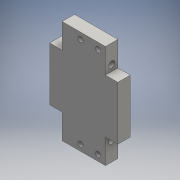
# Autodesk Inventor part: frameBack
Saved by Autodesk Inventor 2016 (Build 200138000, 138)
## iProperties
Created: 2016-05-21
Part Number: frameBack
Material: Generic
Document SubType Name: Modeling
Designer: Henrik Samuelsson
Density: 1 g/cm^3
Appearance: Default
Author: Henrik Samuelsson
Autodesk Inventor part; units mm, degrees
ref_plane "YZ Plane" through (0, 0, 0) normal (1, 0, 0) x (0, 1, 0)
ref_plane "XZ Plane" through (0, 0, 0) normal (0, 1, 0) x (-1, 0, 0)
ref_plane "XY Plane" through (0, 0, 0) normal (0, 0, 1) x (1, 0, 0)
sketch "Sketch1" plane through (0, 0, 0) normal (0, 1, 0) x (-1, 0, 0)
  line L0 (0, 0) -> (66, 0)
  line L1 (66, 0) -> (66, -100)
  line L2 (66, -100) -> (0, -100)
  line L3 (0, -100) -> (0, 0)
  line L4 (66, 0) -> (54, 0)
  line L5 (54, 0) -> (54, -12)
  line L6 (54, -12) -> (66, -12)
  line L7 (66, -12) -> (66, 0)
  line L8 (0, 0) -> (12, 0)
  line L9 (12, 0) -> (12, -12)
  line L10 (12, -12) -> (0, -12)
  line L11 (0, -12) -> (0, 0)
  line L12 (0, -100) -> (12, -100)
  line L13 (12, -100) -> (12, -88)
  line L14 (12, -88) -> (0, -88)
  line L15 (0, -88) -> (0, -100)
  line L16 (66, -100) -> (54, -100)
  line L17 (54, -100) -> (54, -88)
  line L18 (54, -88) -> (66, -88)
  line L19 (66, -88) -> (66, -100)
  dimension "d0" = 66
  dimension "d1" = 100
  dimension "d2" = 12
  dimension "d3" = 12
  dimension "d4" = 12
  dimension "d5" = 12
  dimension "d6" = 12
  dimension "d7" = 12
  dimension "d8" = 12
  dimension "d9" = 12
  constraints: 40 end point, 10 parallel, 5 horizontal, 5 perpendicular
  measures "d0" distance of L1.end L2.end
  measures "d1" distance of L0.end L1.end
  measures "d2" distance of L6.end L5.end
  measures "d3" distance of L5.end L4.end
  measures "d4" distance of L9.end L10.end
  measures "d5" distance of L8.end L9.end
  measures "d6" distance of L14.end L13.end
  measures "d7" distance of L13.end L12.end
  measures "d8" distance of L17.end L18.end
  measures "d9" distance of L16.end L17.end
extrude "Extrusion1" add sketch "Sketch1" along normal blind 12 contours L0 L5 L6 L1 L18 L17 L2 L13 L14 L3 L10 L9
sketch "Sketch5" plane through (-66, 0, -88) normal (-1, 0, 0) x (0, 0, 1)
  line L0 (0, 12) -> (-12, 12) projected
  line L1 (0, 12) -> (12, 12)
  line L2 (12, 12) -> (12, 0)
  line L3 (12, 0) -> (0, 0)
  line L4 (0, 0) -> (0, 12)
  line L5 (76, 12) -> (64, 12)
  line L6 (64, 12) -> (64, 0)
  line L7 (64, 0) -> (76, 0)
  line L8 (76, 0) -> (76, 12)
  point P0 (88, 0)
  dimension "d42" = 12
  dimension "d43" = 12
  dimension "d44" = 12
  dimension "d45" = 12
  dimension "d46" = 12
  constraints: 16 end point, 4 parallel, 2 horizontal, 2 perpendicular, 1 point on line
  measures "d42" distance of L2.end L3.end
  measures "d43" distance of L1.end L2.end
  measures "d44" distance of L7.end L6.end
  measures "d45" distance of L6.end L5.end
  measures "d46" distance of L7.end point (88, 0)
extrude "Extrusion5" cut sketch "Sketch5" against normal blind 12
sketch "Sketch6" plane through (0, 0, -12) normal (1, 0, 0) x (0, 0, -1)
  line L0 (76, 0) -> (76, 12) projected
  line L1 (64, 12) -> (12, 12) projected
  line L2 (76, 0) -> (64, 0)
  line L3 (64, 0) -> (64, 12)
  line L4 (64, 12) -> (76, 12)
  line L5 (76, 12) -> (76, 0)
  line L6 (64, 0) -> (12, 0) projected
  line L7 (12, 12) -> (-12, 12) projected
  line L8 (0, 0) -> (12, 0)
  line L9 (12, 0) -> (12, 12)
  line L10 (12, 12) -> (0, 12)
  line L11 (0, 12) -> (0, 0)
  point P0 (-12, 0)
  dimension "d49" = 12
  dimension "d50" = 12
  constraints: 16 end point, 4 parallel, 2 horizontal, 2 perpendicular
  measures "d49" distance of L1.start L4.end
  measures "d50" distance of L2.end L1.start
extrude "Extrusion6" cut sketch "Sketch6" against normal blind 12 contours L2 L3 L4 L0 | L8 L11 L7 L9
sketch "Sketch7" plane through (-12, -12, -100) normal (1, 0, 0) x (0, 0, -1)
  circle A0 centre (-18, 18) radius 3
  circle A1 centre (-82, 18) radius 3
  line L0 (-100, 24) -> (-76, 24) projected
  line L1 (-76, 24) -> (-76, 12) projected
  line L2 (-24, 12) -> (-24, 24) projected
  line L3 (-24, 24) -> (0, 24) projected
  point P0 (-100, 12)
  dimension "d53" = 6
  dimension "d54" = 6
  dimension "d55" = 6
  dimension "d56" = 6
  dimension "d57" = 6
  dimension "d58" = 6
  constraints: 2 centre point
  measures "d53" diameter of A0
  measures "d54" diameter of A1
  measures "d55" distance from line of L0 A1.centre
  measures "d56" distance from line of L1 A1.centre
  measures "d57" distance from line of L2 A0.centre
  measures "d58" distance from line of L3 A0.centre
extrude "Extrusion7" cut sketch "Sketch7" against normal up to next
sketch "Sketch8" plane through (0, 0, 0) normal (0, -1, 0) x (1, 0, 0)
  circle A0 centre (-19, -6) radius 2.5
  circle A1 centre (-36, -6) radius 2.5
  circle A2 centre (-19, -94) radius 2.5
  circle A3 centre (-36, -94) radius 2.5
  line L0 (-12, -100) -> (-54, -100) projected
  line L1 (-54, 0) -> (-12, 0) projected
  line L2 (-12, 0) -> (-12, -24) projected
  line L3 (-12, -100) -> (-12, -76) projected
  point P0 (0, 0)
  dimension "d61" = 5
  dimension "d62" = 5
  dimension "d63" = 5
  dimension "d64" = 6
  dimension "d65" = 5
  dimension "d66" = 6
  dimension "d67" = 6
  dimension "d68" = 6
  dimension "d69" = 7
  dimension "d70" = 17
  dimension "d71" = 7
  dimension "d72" = 17
  constraints: 4 centre point
  measures "d61" diameter of A1
  measures "d62" diameter of A0
  measures "d63" diameter of A2
  measures "d64" distance from line of L0 A3.centre
  measures "d65" diameter of A3
  measures "d66" distance from line of L0 A2.centre
  measures "d67" distance from line of L1 A0.centre
  measures "d68" distance from line of L1 A1.centre
  measures "d69" distance from line of L2 A0.centre
  measures "d70" distance of A1.centre A0.centre
  measures "d71" distance from line of A2.centre L3
  measures "d72" distance of A3.centre A2.centre
extrude "Extrusion8" cut sketch "Sketch8" against normal blind 6
fillet "Fillet1" radius 2.5 4 edges at (-21.5, 6, -6) (-38.5, 6, -6) (-38.5, 6, -94) (-21.5, 6, -94)
body "Solid1"
